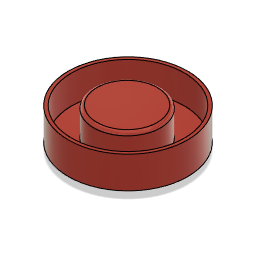
Fan_AVC_BASA0725R2U v3 (Autodesk Fusion 360 design; units mm, degrees)
Autodesk Fusion 360 part; units mm, degrees
sketch "Sketch1" plane through (0, 0, 0) normal (0, 1, 0) x (1, 0, 0)
  circle A0 centre (0, 0) radius 21.362
  line L0 (0, 0) -> (21.362, 0)
  circle A1 centre (21.362, 0) radius 1.25
  circle A2 centre (-10.681, 18.5) radius 1.25
  circle A3 centre (-10.681, -18.5) radius 1.25
  line L1 (-10.681, 18.5) -> (21.362, 0) construction
  line L2 (-14.1333, 19.2835) -> (-14.1333, -19.2835)
  line L3 (-9.6333, -21.8816) -> (23.7667, -2.5981)
  line L4 (23.7667, 2.5981) -> (-9.6333, 21.8816)
  line L5 (-14.1333, 24.4797) -> (7.0667, -12.2398) construction
  line L6 (28.2667, 0) -> (-14.1333, 0) construction
  line L7 (-14.1333, -24.4797) -> (7.0667, 12.2398) construction
  arc A4 (-9.6333, 21.8816) -> (-14.1333, 19.2835) centre (-11.1333, 19.2835) ccw
  arc A5 (23.7667, -2.5981) -> (23.7667, 2.5981) centre (22.2667, 0) ccw
  arc A6 (-14.1333, -19.2835) -> (-9.6333, -21.8816) centre (-11.1333, -19.2835) ccw
  line L8 (25.2667, 13) -> (25.2667, -18) construction
  line L9 (-14.1333, -5) -> (-24.1333, -5)
  line L10 (-24.1333, -5) -> (-24.1333, 5)
  line L11 (-24.1333, 5) -> (-14.1333, 5)
  line L12 (-14.1333, 5) -> (-14.1333, -5)
  line L13 (-14.1333, -5) -> (-24.1333, 5) construction
  line L14 (-24.1333, -5) -> (-14.1333, 5) construction
  point P0 (-19.1333, 0)
  dimension "d1" = 2.5
  dimension "d3" = 360
  dimension "d4" = 37
  dimension "d6" = 60
  dimension "d7" = 60
  dimension "d8" = 3
  dimension "d9" = 39.4
  dimension "d12" = 10
  dimension "d13" = 10
  constraint coincident A0.centre L0.start
  constraint coincident A0 L0.end
  constraint horizontal L0
  constraint coincident L0.end A1.centre
  constraint coincident A2.centre L1.start
  constraint vertical L2
  constraint coincident L3 L5.end
  constraint perpendicular L3 L5
  constraint coincident L2 L6.end
  constraint perpendicular L2 L6
  constraint coincident L4 L7.end
  constraint perpendicular L4 L7
  constraint coincident L7 A0.centre
  constraint coincident L5 A0.centre
  constraint coincident L2 L5.start
  constraint coincident L5.start L4
  constraint tangent L2 A4
  constraint tangent L4 A4
  constraint coincident L6.start L4
  constraint coincident L6.start L3
  constraint tangent L4 A5
  constraint tangent L3 A5
  constraint equal A4 A5
  constraint coincident L7.start L3
  constraint coincident L7.start L2
  constraint tangent L3 A6
  constraint tangent L2 A6
  constraint equal A4 A6
  constraint vertical L8
  constraint tangent A5 L8
  constraint horizontal L9
  constraint perpendicular L9 L10
  constraint parallel L9 L11
  constraint parallel L10 L12
  constraint coincident L2 L9.start
  constraint coincident L13 P0
  constraint coincident L14 P0
  measures "d1" diameter of A1
  measures "d4" distance of A2.centre L0.end
  measures "d6" angle of L2 L3
  measures "d7" angle of L2 L4
  measures "d8" radius of A4
  measures "d9" distance of L2 L8
  measures "d12" distance of L9.start L9.end
  measures "d13" distance of L9.end L10.end
extrude "Extrude1" add sketch "Sketch1" along normal blind 1.2 contours A0 A1 A2 A3 L2 L3 L4 L12 | A0 A1 L3 L4 A5 | A0 A2 L2 L4 A4 | A0 A3 L2 L3 A6 | A0 L2 L9 L11 L12 | A0 L9 L10 L11 makes body 1
ref_plane "WorkPlane1" through (0.5667, 4.5, 0) normal (0, 1, 0) x (1, 0, 0)
sketch "Sketch2" plane through (0.5667, 4.5, 0) normal (0, 1, 0) x (1, 0, 0)
  circle A0 centre (0, 0) radius 37.5
  dimension "d15" = 75
  constraint coincident A0.centre origin
  measures "d15" diameter of A0
extrude "Extrude2" add sketch "Sketch2" along normal blind 20 separate body makes body 2
shell "Shell1" thickness 2 removed faces 1 at (5.273, 24.5, -13.499) on bodies 2
sketch "Sketch3" plane through (0, 6.5, 0) normal (0, 1, 0) x (-1, 0, 0)
  circle A0 centre (-0.5667, 0) radius 35.5
  circle A1 centre (0, 0) radius 21
  dimension "d19" = 42
  constraint coincident A1.centre origin
  measures "d19" diameter of A1
extrude "Extrude3" add sketch "Sketch3" along normal up to surface (18 mm away) contours A1 bodies 2
fillet "Fillet1" radius 2 1 edges at (19.5789, 24.5, 7.5939) on bodies 2
